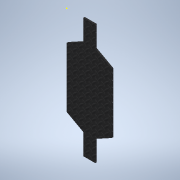
# Autodesk Inventor part: Base_plate_2
Saved by Autodesk Inventor 2020 (Build 240168000, 168)
## iProperties
Created: 2015-12-01
Part Number: Base_plate_2
Material: Polímero reforzado con fibra de carbono
Document SubType Name: Modeling
Designer: MIGUEL ANGEL
Density: 1.43 g/cm^3
Appearance: Placa de rombos 2 - Gris oscuro
Author: MIGUEL ANGEL
Autodesk Inventor part; units mm, degrees
ref_plane "XZ Plane" through (0, 0, 0) normal (0, 1, 0) x (-1, 0, 0)
ref_plane "XY Plane" through (0, 0, 0) normal (0, 0, 1) x (1, 0, 0)
sketch "Boceto1" plane through (0, 0, 0) normal (0, 1, 0) x (-1, 0, 0)
  line L0 (0, 0) -> (-300, 0)
  line L1 (-300, 0) -> (-300, -800)
  line L2 (-300, -800) -> (0, -800)
  line L3 (0, -800) -> (0, 0)
  dimension "d0" = 800
  dimension "d1" = 300
  constraints: 8 end point, 2 parallel, 1 horizontal, 1 perpendicular
  measures "d0" distance of L0.end L1.end
  measures "d1" distance of L1.end L2.end
extrude "Extrusión1" add sketch "Boceto1" along normal blind 20
sketch "Boceto2" plane through (0, 20, 0) normal (0, 1, 0) x (1, 0, 0)
  line L0 (0, 800) -> (0, 0) projected
  line L1 (300, 0) -> (300, 800) projected
  line L2 (0, 0) -> (300, 0) projected
  line L3 (300, 800) -> (0, 800) projected
  line L4 (0, 200) -> (110, 140)
  line L5 (110, 140) -> (110, 65.0388)
  line L6 (110, 65.0388) -> (110, 0)
  line L7 (110, 800) -> (110, 725.0388)
  line L8 (110, 725.0388) -> (110, 660)
  line L9 (0, 600) -> (110, 660)
  line L10 (150, -80.8497) -> (150, 1003.0293) construction
  line L11 (-90.141, 400) -> (345.1137, 400) construction
  line L12 (190, 0) -> (190, 140)
  line L13 (190, 140) -> (300, 200)
  line L14 (300, 600) -> (190, 660)
  line L15 (190, 660) -> (190, 800)
  line L16 (110, 40) -> (95, 44.2247)
  arc A0 (95, 55.7753) -> (95, 44.2247) centre (96.6266, 50) ccw
  line L17 (95, 55.7753) -> (110, 60)
  line L18 (190, 40) -> (205, 44.2247)
  arc A1 (205, 44.2247) -> (205, 55.7753) centre (203.3734, 50) ccw
  line L19 (205, 55.7753) -> (190, 60)
  line L20 (110, 760) -> (95, 755.7753)
  arc A2 (95, 755.7753) -> (95, 744.2247) centre (96.6266, 750) ccw
  line L21 (95, 744.2247) -> (110, 740)
  line L22 (205, 744.2247) -> (190, 740)
  arc A3 (205, 744.2247) -> (205, 755.7753) centre (203.3734, 750) ccw
  line L23 (190, 760) -> (205, 755.7753)
  line L24 (110, 40) -> (110, 60)
  line L25 (190, 40) -> (190, 60)
  line L26 (110, 740) -> (110, 760)
  line L27 (190, 740) -> (190, 760)
  dimension "d4" = 110
  dimension "d5" = 150
  dimension "d7" = 140
  dimension "d8" = 200
  dimension "d9" = 400
  dimension "d12" = 15
  dimension "d13" = 6
  dimension "d14" = 20
  dimension "d15" = 40
  constraints: 49 end point, 15 symmetric about line, 12 point on line, 8 point on circle, 4 centre point, 4 collinear, 4 equal length, 4 vertical, 2 tangent, 1 horizontal, 1 horizontal alignment, 1 perpendicular, 7 other
  measures "d4" distance between parallel lines of L0 L5
  measures "d5" distance between parallel lines of L10 L1
  measures "d7" distance of L4.end L6.end
  measures "d8" distance of L0.end L4.start
  measures "d9" distance between parallel lines of L2 L11
  measures "d12" horizontal distance of L16.start L16.end
  measures "d13" radius of A0
  measures "d14" distance of L17.end L16.start
  measures "d15" distance of L16.start L6.end
extrude "Extrusión2" cut sketch "Boceto2" against normal through all contours L3 L7 L20 A2 L21 L8 L9 L0 | L4 L5 L6 L17 A0 L16 L2 L0 | L3 L1 L14 L15 L22 A3 L23 | L7 L21 A2 L20 | L23 A3 L22 L15 | L12 L18 A1 L19 L13 L1 L2 | L16 A0 L17 L6 | L12 L19 A1 L18
extrude "Extrusión3" cut sketch "Boceto1" along normal blind 10
ref_plane "Plano de trabajo1" through (150, 0, 0) normal (1, 0, 0) x (0, 1, 0)
sketch "Boceto8" plane through (0, 10, 0) normal (0, -1, 0) x (1, 0, 0)
  point P0 (0, 0)
sketch "Boceto9" plane through (0, 20, 0) normal (0, 1, 0) x (1, 0, 0)
  point P0 (284, 300)
hole "Agujero1" at (284, 20, -300) direction (0, -1, 0) diameter 3.7973 depth 10
sketch "Boceto10" plane through (0, 20, 0) normal (0, 1, 0) x (1, 0, 0)
  point P0 (190, 300)
hole "Agujero3" at (190, 20, -300) direction (0, -1, 0) diameter 3.7973 depth 10
sketch "Boceto11" plane through (0, 20, 0) normal (0, 1, 0) x (1, 0, 0)
  point P0 (183.5, 23)
hole "Agujero5" at (183.5, 20, -23) direction (0, -1, 0) diameter 3.7973 depth 10
sketch "Boceto12" plane through (0, 20, 0) normal (0, 1, 0) x (1, 0, 0)
  point P0 (118.5, 23)
hole "Agujero7" at (118.5, 20, -23) direction (0, -1, 0) diameter 3.7973 depth 10
sketch "Boceto13" plane through (0, 20, 0) normal (0, 1, 0) x (1, 0, 0)
  point P0 (118.745, 107)
hole "Agujero9" at (118.745, 20, -107) direction (0, -1, 0) diameter 3.7973 depth 10
sketch "Boceto14" plane through (0, 20, 0) normal (0, 1, 0) x (1, 0, 0)
  point P0 (183.745, 107)
hole "Agujero11" at (183.745, 20, -107) direction (0, -1, 0) diameter 3.7973 depth 10
sketch "Boceto15" plane through (0, 20, 0) normal (0, 1, 0) x (1, 0, 0)
  point P0 (117.3, 777)
hole "Agujero13" at (117.3, 20, -777) direction (0, -1, 0) diameter 3.7973 depth 10
sketch "Boceto16" plane through (0, 20, 0) normal (0, 1, 0) x (1, 0, 0)
  point P0 (181.9092, 693)
hole "Agujero15" at (181.9092, 20, -693) direction (0, -1, 0) diameter 3.7973 depth 10
sketch "Boceto17" plane through (0, 20, 0) normal (0, 1, 0) x (1, 0, 0)
  point P0 (116.9092, 693)
hole "Agujero17" at (116.9092, 20, -693) direction (0, -1, 0) diameter 3.7973 depth 10
sketch "Boceto18" plane through (0, 20, 0) normal (0, 1, 0) x (1, 0, 0)
  point P0 (182.3, 777)
hole "Agujero19" at (182.3, 20, -777) direction (0, -1, 0) diameter 3.7973 depth 10
